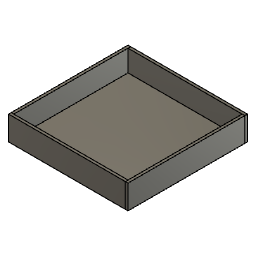
ParametricMold (Autodesk Fusion 360 design; units mm, degrees)
Autodesk Fusion 360 part; units mm, degrees
sketch "Sketch1" plane through (0, 0, 0) normal (0, 1, 0) x (1, 0, 0)
  line L0 (0, 0) -> (812.8, 0)
  line L1 (812.8, 0) -> (812.8, -812.8)
  line L2 (812.8, -812.8) -> (0, -812.8)
  line L3 (0, -812.8) -> (0, 0)
  line L4 (0, 0) -> (831.596, 0)
  line L5 (831.596, 0) -> (831.596, 18.796)
  line L6 (831.596, 18.796) -> (0, 18.796)
  line L7 (0, 18.796) -> (0, 0)
  line L8 (812.8, 0) -> (831.596, 0)
  line L9 (831.596, 0) -> (831.596, -831.596)
  line L10 (831.596, -831.596) -> (812.8, -831.596)
  line L11 (812.8, -831.596) -> (812.8, 0)
  line L12 (812.8, -831.596) -> (-18.796, -831.596)
  line L13 (-18.796, -831.596) -> (-18.796, -812.8)
  line L14 (-18.796, -812.8) -> (812.8, -812.8)
  line L15 (812.8, -812.8) -> (812.8, -831.596)
  line L16 (-18.796, -812.8) -> (0, -812.8)
  line L17 (0, -812.8) -> (0, 18.796)
  line L18 (0, 18.796) -> (-18.796, 18.796)
  line L19 (-18.796, 18.796) -> (-18.796, -812.8)
  dimension "d5" = 812.8
  dimension "d6" = 812.8
  dimension "d7" = 831.596
  dimension "d8" = 18.796
  dimension "d9" = 18.796
  dimension "d10" = 831.596
  dimension "d11" = 831.596
  dimension "d12" = 18.796
  dimension "d13" = 18.796
  dimension "d14" = 831.596
  constraint horizontal L0
  constraint vertical L1
  constraint horizontal L2
  constraint vertical L3
  constraint coincident L0.start L3.end
  constraint horizontal L4
  constraint vertical L5
  constraint horizontal L6
  constraint vertical L7
  constraint horizontal L8
  constraint vertical L9
  constraint horizontal L10
  constraint vertical L11
  constraint horizontal L12
  constraint vertical L13
  constraint horizontal L14
  constraint vertical L15
  constraint horizontal L16
  constraint vertical L17
  constraint horizontal L18
  constraint vertical L19
  measures "d5" distance of L0.start L0.end
  measures "d6" distance of L0.start L2.end
  measures "d7" distance of L0.start L4.end
  measures "d8" distance of L0.start L6.end
  measures "d9" distance of L0.end L4.end
  measures "d10" distance of L0.end L10.end
  measures "d11" distance of L10.end L12.end
  measures "d12" distance of L10.end L1.end
  measures "d13" distance of L13.end L2.end
  measures "d14" distance of L13.end L18.end
extrude "Extrude1" add sketch "Sketch1" along normal blind 18.796 contours L0 L1 L2 L3 L4 L11 L14 L17 makes body 1 in component "Base"
extrude "Extrude1'" add sketch "Sketch1" along normal blind 171.196 separate body contours L0 L4 L5 L6 L7 L8 L17 makes body 2 in component "width1"
extrude "Extrude1''" add sketch "Sketch1" along normal blind 171.196 separate body contours L3 L7 L14 L16 L17 L18 L19 makes body 3 in component "length1"
extrude "Extrude1'''" add sketch "Sketch1" along normal blind 171.196 separate body contours L2 L11 L12 L13 L14 L15 L16 makes body 4 in component "width2"
extrude "Extrude1''''" add sketch "Sketch1" along normal blind 171.196 separate body contours L1 L4 L8 L9 L10 L11 L15 makes body 5 in component "length2"
component "Base" placed x (1, 0, 0) y (0, 1, 0) z (0, 0, 1) at (0, 0, 0)
component "width1" placed x (1, 0, 0) y (0, 1, 0) z (0, 0, 1) at (0, 0, 0)
component "length1" placed x (1, 0, 0) y (0, 1, 0) z (0, 0, 1) at (0, 0, 0)
component "width2" placed x (1, 0, 0) y (0, 1, 0) z (0, 0, 1) at (0, 0, 0)
component "length2" placed x (1, 0, 0) y (0, 1, 0) z (0, 0, 1) at (0, 0, 0)
equation "projectWidth = 32 in"
equation "projectLength = 32 in"
equation "materialThickness = 0.74 in"
equation "pourThickness = 5 in + materialThickness + headroom"
equation "d5 = projectWidth"
equation "d6 = projectLength"
equation "d7 = projectWidth + materialThickness"
equation "d8 = materialThickness"
equation "d9 = materialThickness"
equation "d10 = projectLength + materialThickness"
equation "d11 = projectWidth + materialThickness"
equation "d12 = materialThickness"
equation "d13 = materialThickness"
equation "d14 = projectLength + materialThickness"
equation "d15 = materialThickness"
equation "d17 = pourThickness"
equation "d19 = pourThickness"
equation "d21 = pourThickness"
equation "d23 = pourThickness"
equation "headroom = 1 in"
